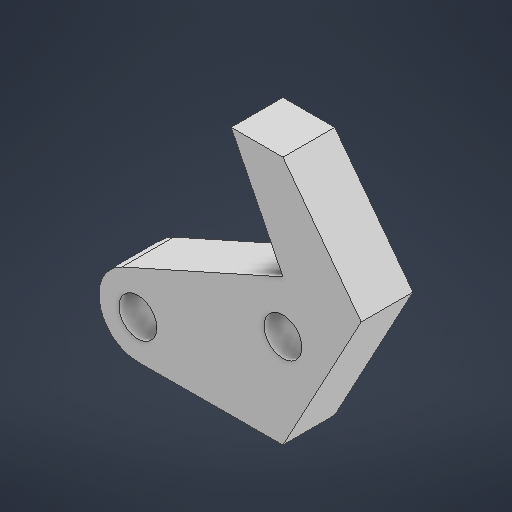
# Autodesk Inventor part: Goal Jaw Tooth
Saved by Autodesk Inventor 2025 (Build 290162000, 162)
## iProperties
Created: 2025-02-08
Part Number: Goal Jaw Tooth
Material: Generic
Document SubType Name: Modeling
Designer: Juan
Density: 1 g/cm^3
Appearance: Default
Author: Juan
Autodesk Inventor part; units mm, degrees
ref_plane "YZ Plane" through (0, 0, 0) normal (1, 0, 0) x (0, 1, 0)
ref_plane "XZ Plane" through (0, 0, 0) normal (0, 1, 0) x (-1, 0, 0)
ref_plane "XY Plane" through (0, 0, 0) normal (0, 0, 1) x (1, 0, 0)
sketch "Sketch1" plane through (0, 0, 0) normal (0, 0, 1) x (1, 0, 0)
  circle A0 centre (0, 0) radius 2.3241
  circle A1 centre (0, 0) radius 11.5062
  line L0 (0, 0) -> (0, 6.35)
  line L1 (0, 6.35) -> (1.4708, 6.35)
  line L2 (1.4708, 6.35) -> (9.5953, 6.35)
  line L3 (0, 6.35) -> (0, 19.05)
  line L4 (0, 19.05) -> (-6.35, 19.05)
  line L5 (-6.35, 19.05) -> (0, 6.35)
  line L6 (9.5953, 6.35) -> (0, 19.05)
  line L7 (0, 6.35) -> (-35.4663, 6.35)
  circle A2 centre (0, 0) radius 19.05
  line L8 (-30.5707, -30.0948) -> (-7.7493, -41.2459)
  circle A3 centre (4.7977, -18.436) radius 2.3241
  circle A4 centre (4.7977, -18.436) radius 4.7625
  line L9 (4.7977, -18.436) -> (-17.7887, -6.8164)
  circle A5 centre (-17.7887, -6.8164) radius 2.3241
  circle A6 centre (-17.7887, -6.8164) radius 4.7625
  line L10 (0, 6.35) -> (-19.7319, -2.4684)
  line L11 (9.5953, 6.35) -> (0, -11.5062)
  line L12 (0, -11.5062) -> (-17.7693, -11.5789)
  dimension "d0" = 4.6482
  dimension "d1" = 23.0124
  dimension "d2" = 6.35
  dimension "d3" = 12.7
  dimension "d4" = 6.35
  dimension "d5" = 25.4
  dimension "d6" = 4.6482
  dimension "d7" = 9.525
  dimension "d8" = 25.4
  dimension "d9" = 4.6482
  dimension "d10" = 9.525
  constraints: 26 end point, 7 centre point, 7 point on circle, 6 coincident, 2 point on line, 2 tangent, 1 horizontal, 1 perpendicular, 1 vertical
  measures "d0" diameter of A0
  measures "d1" diameter of A1
  measures "d2" distance of L0.start L0.end
  measures "d3" distance of L0.end L3.end
  measures "d4" distance of L3.end L4.end
  measures "d5" distance of L8.start L8.end
  measures "d6" diameter of A3
  measures "d7" diameter of A4
  measures "d8" distance of L9.start L9.end
  measures "d9" diameter of A5
  measures "d10" diameter of A6
extrude "Extrusion1" add sketch "Sketch1" along normal blind 6.35 contours L1 L2 L11 A1 L10 | L5 A1 L3 | L3 A1 L6 L2 L1 | L3 L6 A1 | A1 L5 A2 L3 | A1 L12 L9 A6 A2 L10 | A2 L5 L4 | A2 A6 L10 | L12 A2 A6 L9 | A6 L9 A5 A2 | A2 A5 A6 | A6 A2 A5 L9 | L12 A6 A2
body "Solid1"
